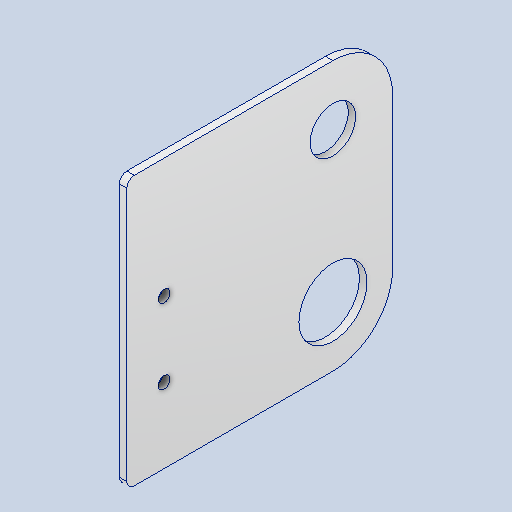
# Autodesk Inventor part: dribl-v1-Plate-5
Saved by Autodesk Inventor 2025.2 (Build 292293000, 293)
## iProperties
Created: 2025-01-07
Part Number: dribl-v1-Plate-5
Material: アルミニウム 6061
Document SubType Name: Modeling
Designer: haruy
Density: 2.7 g/cm^3
Appearance: アルミニウム - フラット
Author: haruy
Autodesk Inventor part; units mm, degrees
ref_plane "YZ Plane" through (0, 0, 0) normal (1, 0, 0) x (0, 1, 0)
ref_plane "XZ Plane" through (0, 0, 0) normal (0, 1, 0) x (-1, 0, 0)
ref_plane "XY Plane" through (0, 0, 0) normal (0, 0, 1) x (1, 0, 0)
derived "dribl-v1-ASP-Base.ipt"
sketch "スケッチ5" plane through (-210, -432.3334, -303) normal (-1, 0, 0) x (0, 0, 1)
  circle A0 centre (-55.18, 231) radius 16 projected
  line L0 (-20, 0) -> (-20, 1308) projected
  circle A1 centre (-55.18, 191) radius 16 projected
  line L1 (-20, 82) -> (-319.0594, 82) projected
  line L2 (-319.0594, 82) -> (-319.0594, 102) projected
  line L3 (-319.0594, 102) -> (-20, 102) projected
  line L4 (-20, 102) -> (-20, 82) projected
  line L5 (0, 0) -> (-20, 0) projected
  circle A2 centre (-55.18, 191) radius 9.1 projected
  line L6 (-55.18, 247) -> (0, 247) projected
  line L7 (-71.18, 231) -> (-71.18, 191) projected
  line L8 (-55.18, 175) -> (0, 175) projected
  line L9 (0, 1308) -> (0, 0) projected
  circle A3 centre (-10, 215) radius 1.6 projected
  circle A4 centre (-10, 195) radius 1.6 projected
  circle A5 centre (-55.18, 231) radius 6.1 projected
  point P0 (303, 432.3334)
  point P1 (-169.5297, 102)
extrude "押し出し1" add sketch "スケッチ5" against normal blind 2 contours A0 | A0 L6 L0 L8 A1 L7 | L6 L9 L8 L0 | A1
fillet "フィレット1" radius 2 2 edges at (-209, -185.3334, -303) (-209, -257.3334, -303)
